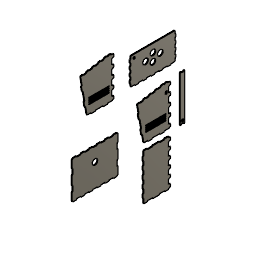
FINAL_CONSOLE (Autodesk Fusion 360 design; units mm, degrees)
part number: 2026-05-18-11-19-14-650
Autodesk Fusion 360 part; units mm, degrees
(part 1 of 2)
sketch "Sketch1" plane through (0, 0, 0) normal (1, 0, 0) x (0, 1, 0)
  line L0 (-1580.457, 35.3013) -> (-1610.457, 35.3013) construction
  line L1 (-1670.457, -232.1266) -> (-1670.457, -238.1266)
  line L2 (-1610.457, 43.2364) -> (-1580.457, 43.2364)
  line L3 (-1580.457, -232.1266) -> (-1574.457, -232.1266)
  line L4 (-1580.457, -22.7636) -> (-1574.457, -22.7636)
  line L5 (-1580.457, -232.1266) -> (-1580.457, 37.2364)
  line L6 (-1610.457, 37.2364) -> (-1610.457, 43.2364)
  line L7 (-1670.457, -238.1266) -> (-1640.457, -238.1266)
  line L8 (-1574.457, -232.1266) -> (-1574.457, -172.1266)
  line L9 (-1610.457, -232.1266) -> (-1610.457, -238.1266)
  line L10 (-1760.457, -232.1266) -> (-1760.457, -238.1266)
  line L11 (-1910.457, -232.1266) -> (-1580.457, -232.1266)
  line L12 (-1760.457, 43.2364) -> (-1790.457, 43.2364)
  line L13 (-1910.457, -232.1266) -> (-1580.457, -232.1266)
  line L14 (-1730.457, 37.2364) -> (-1730.457, 43.2364)
  line L15 (-1790.457, -238.1266) -> (-1760.457, -238.1266)
  line L16 (-1910.457, -232.1266) -> (-1580.457, -232.1266)
  line L17 (-1910.457, -232.1266) -> (-1580.457, -232.1266)
  circle A0 centre (-1745.457, -62.7636) radius 20
  line L18 (-1580.457, 37.2364) -> (-1910.457, 37.2364)
  line L19 (-1910.457, 37.2364) -> (-1910.457, -232.1266)
  line L20 (-1910.457, -172.1266) -> (-1916.457, -172.1266)
  line L21 (-1916.457, -22.7636) -> (-1916.457, 37.2364)
  line L22 (-1910.457, -22.7636) -> (-1916.457, -22.7636)
  line L23 (-1820.457, 37.2364) -> (-1820.457, 43.2364)
  line L24 (-1916.457, -132.1266) -> (-1916.457, -62.7636)
  line L25 (-1850.457, -232.1266) -> (-1850.457, -238.1266)
  line L26 (-1910.457, -238.1266) -> (-1880.457, -238.1266)
  line L27 (-1910.457, 37.2364) -> (-1910.457, 43.2364)
  line L28 (-1910.457, -62.7636) -> (-1916.457, -62.7636)
  line L29 (-1910.457, -232.1266) -> (-1910.457, -238.1266)
  line L30 (-1910.457, 43.2364) -> (-1880.457, 43.2364)
  line L31 (-1610.457, -238.1266) -> (-1580.457, -238.1266)
  line L32 (-1640.457, -232.1266) -> (-1640.457, -238.1266)
  line L33 (-1640.457, 43.2364) -> (-1670.457, 43.2364)
  line L34 (-1580.457, -232.1266) -> (-1580.457, -238.1266)
  line L35 (-1670.457, 37.2364) -> (-1670.457, 43.2364)
  line L36 (-1760.457, 37.2364) -> (-1760.457, 43.2364)
  line L37 (-1580.457, -172.1266) -> (-1574.457, -172.1266)
  line L38 (-1574.457, -132.1266) -> (-1574.457, -62.7636)
  line L39 (-1640.457, 37.2364) -> (-1640.457, 43.2364)
  line L40 (-1820.457, -232.1266) -> (-1820.457, -238.1266)
  line L41 (-1700.457, 43.2364) -> (-1730.457, 43.2364)
  line L42 (-1700.457, 37.2364) -> (-1700.457, 43.2364)
  line L43 (-1574.457, -22.7636) -> (-1574.457, 37.2364)
  line L44 (-1700.457, -232.1266) -> (-1700.457, -238.1266)
  line L45 (-1580.457, 37.2364) -> (-1574.457, 37.2364)
  line L46 (-1580.457, 37.2364) -> (-1580.457, 43.2364)
  line L47 (-1580.457, -132.1266) -> (-1574.457, -132.1266)
  line L48 (-1730.457, -232.1266) -> (-1730.457, -238.1266)
  line L49 (-1730.457, -238.1266) -> (-1700.457, -238.1266)
  line L50 (-1850.457, -238.1266) -> (-1820.457, -238.1266)
  line L51 (-1580.457, -62.7636) -> (-1574.457, -62.7636)
  line L52 (-1916.457, -232.1266) -> (-1916.457, -172.1266)
  line L53 (-1880.457, 43.2364) -> (-1880.457, 37.2364)
  line L54 (-1910.457, -232.1266) -> (-1916.457, -232.1266)
  line L55 (-1790.457, -232.1266) -> (-1790.457, -238.1266)
  line L56 (-1910.457, 37.2364) -> (-1916.457, 37.2364)
  line L57 (-1820.457, 43.2364) -> (-1850.457, 43.2364)
  line L58 (-1880.457, -232.1266) -> (-1880.457, -238.1266)
  line L59 (-1850.457, 37.2364) -> (-1850.457, 43.2364)
  line L60 (-1790.457, 37.2364) -> (-1790.457, 43.2364)
  line L61 (-1910.457, -132.1266) -> (-1916.457, -132.1266)
  line L62 (-1580.457, 35.3013) -> (-1610.457, 35.3013) construction
  line L63 (-1670.457, -232.1266) -> (-1670.457, -238.1266)
  line L64 (-1610.457, 43.2364) -> (-1580.457, 43.2364)
  line L65 (-1580.457, -232.1266) -> (-1574.457, -232.1266)
  line L66 (-1580.457, -22.7636) -> (-1574.457, -22.7636)
  line L67 (-1580.457, -232.1266) -> (-1580.457, 37.2364)
  line L68 (-1610.457, 37.2364) -> (-1610.457, 43.2364)
  line L69 (-1670.457, -238.1266) -> (-1640.457, -238.1266)
  line L70 (-1574.457, -232.1266) -> (-1574.457, -172.1266)
  line L71 (-1610.457, -232.1266) -> (-1610.457, -238.1266)
  line L72 (-1760.457, -232.1266) -> (-1760.457, -238.1266)
  line L73 (-1910.457, -232.1266) -> (-1580.457, -232.1266)
  line L74 (-1760.457, 43.2364) -> (-1790.457, 43.2364)
  line L75 (-1910.457, -232.1266) -> (-1580.457, -232.1266)
  line L76 (-1730.457, 37.2364) -> (-1730.457, 43.2364)
  line L77 (-1790.457, -238.1266) -> (-1760.457, -238.1266)
  line L78 (-1910.457, -232.1266) -> (-1580.457, -232.1266)
  line L79 (-1910.457, -232.1266) -> (-1580.457, -232.1266)
  circle A1 centre (-1745.457, -62.7636) radius 20
  line L80 (-1580.457, 37.2364) -> (-1910.457, 37.2364)
  line L81 (-1910.457, 37.2364) -> (-1910.457, -232.1266)
  line L82 (-1910.457, -172.1266) -> (-1916.457, -172.1266)
  line L83 (-1916.457, -22.7636) -> (-1916.457, 37.2364)
  line L84 (-1910.457, -22.7636) -> (-1916.457, -22.7636)
  line L85 (-1820.457, 37.2364) -> (-1820.457, 43.2364)
  line L86 (-1916.457, -132.1266) -> (-1916.457, -62.7636)
  line L87 (-1850.457, -232.1266) -> (-1850.457, -238.1266)
  line L88 (-1910.457, -238.1266) -> (-1880.457, -238.1266)
  line L89 (-1910.457, 37.2364) -> (-1910.457, 43.2364)
  line L90 (-1910.457, -62.7636) -> (-1916.457, -62.7636)
  line L91 (-1910.457, -232.1266) -> (-1910.457, -238.1266)
  line L92 (-1910.457, 43.2364) -> (-1880.457, 43.2364)
  line L93 (-1610.457, -238.1266) -> (-1580.457, -238.1266)
  line L94 (-1640.457, -232.1266) -> (-1640.457, -238.1266)
  line L95 (-1640.457, 43.2364) -> (-1670.457, 43.2364)
  line L96 (-1580.457, -232.1266) -> (-1580.457, -238.1266)
  line L97 (-1670.457, 37.2364) -> (-1670.457, 43.2364)
  line L98 (-1760.457, 37.2364) -> (-1760.457, 43.2364)
  line L99 (-1580.457, -172.1266) -> (-1574.457, -172.1266)
  line L100 (-1574.457, -132.1266) -> (-1574.457, -62.7636)
  line L101 (-1640.457, 37.2364) -> (-1640.457, 43.2364)
  line L102 (-1820.457, -232.1266) -> (-1820.457, -238.1266)
  line L103 (-1700.457, 43.2364) -> (-1730.457, 43.2364)
  line L104 (-1700.457, 37.2364) -> (-1700.457, 43.2364)
  line L105 (-1574.457, -22.7636) -> (-1574.457, 37.2364)
  line L106 (-1700.457, -232.1266) -> (-1700.457, -238.1266)
  line L107 (-1580.457, 37.2364) -> (-1574.457, 37.2364)
  line L108 (-1580.457, 37.2364) -> (-1580.457, 43.2364)
  line L109 (-1580.457, -132.1266) -> (-1574.457, -132.1266)
  line L110 (-1730.457, -232.1266) -> (-1730.457, -238.1266)
  line L111 (-1730.457, -238.1266) -> (-1700.457, -238.1266)
  line L112 (-1850.457, -238.1266) -> (-1820.457, -238.1266)
  line L113 (-1580.457, -62.7636) -> (-1574.457, -62.7636)
  line L114 (-1916.457, -232.1266) -> (-1916.457, -172.1266)
  line L115 (-1880.457, 43.2364) -> (-1880.457, 37.2364)
  line L116 (-1910.457, -232.1266) -> (-1916.457, -232.1266)
  line L117 (-1790.457, -232.1266) -> (-1790.457, -238.1266)
  line L118 (-1910.457, 37.2364) -> (-1916.457, 37.2364)
  line L119 (-1820.457, 43.2364) -> (-1850.457, 43.2364)
  line L120 (-1880.457, -232.1266) -> (-1880.457, -238.1266)
  line L121 (-1850.457, 37.2364) -> (-1850.457, 43.2364)
  line L122 (-1790.457, 37.2364) -> (-1790.457, 43.2364)
  line L123 (-1910.457, -132.1266) -> (-1916.457, -132.1266)
  line L124 (-1580.457, 35.3013) -> (-1610.457, 35.3013) construction
  line L125 (-1670.457, -232.1266) -> (-1670.457, -238.1266)
  line L126 (-1610.457, 43.2364) -> (-1580.457, 43.2364)
  line L127 (-1580.457, -232.1266) -> (-1574.457, -232.1266)
  line L128 (-1580.457, -22.7636) -> (-1574.457, -22.7636)
  line L129 (-1580.457, -232.1266) -> (-1580.457, 37.2364)
  line L130 (-1610.457, 37.2364) -> (-1610.457, 43.2364)
  line L131 (-1670.457, -238.1266) -> (-1640.457, -238.1266)
  line L132 (-1574.457, -232.1266) -> (-1574.457, -172.1266)
  line L133 (-1610.457, -232.1266) -> (-1610.457, -238.1266)
  line L134 (-1760.457, -232.1266) -> (-1760.457, -238.1266)
  line L135 (-1910.457, -232.1266) -> (-1580.457, -232.1266)
  line L136 (-1760.457, 43.2364) -> (-1790.457, 43.2364)
  line L137 (-1910.457, -232.1266) -> (-1580.457, -232.1266)
  line L138 (-1730.457, 37.2364) -> (-1730.457, 43.2364)
  line L139 (-1790.457, -238.1266) -> (-1760.457, -238.1266)
  line L140 (-1910.457, -232.1266) -> (-1580.457, -232.1266)
  line L141 (-1910.457, -232.1266) -> (-1580.457, -232.1266)
  circle A2 centre (-1745.457, -62.7636) radius 20
  line L142 (-1580.457, 37.2364) -> (-1910.457, 37.2364)
  line L143 (-1910.457, 37.2364) -> (-1910.457, -232.1266)
  line L144 (-1910.457, -172.1266) -> (-1916.457, -172.1266)
  line L145 (-1916.457, -22.7636) -> (-1916.457, 37.2364)
  line L146 (-1910.457, -22.7636) -> (-1916.457, -22.7636)
  line L147 (-1820.457, 37.2364) -> (-1820.457, 43.2364)
  line L148 (-1916.457, -132.1266) -> (-1916.457, -62.7636)
  line L149 (-1850.457, -232.1266) -> (-1850.457, -238.1266)
  line L150 (-1910.457, -238.1266) -> (-1880.457, -238.1266)
  line L151 (-1910.457, 37.2364) -> (-1910.457, 43.2364)
  line L152 (-1910.457, -62.7636) -> (-1916.457, -62.7636)
  line L153 (-1910.457, -232.1266) -> (-1910.457, -238.1266)
  line L154 (-1910.457, 43.2364) -> (-1880.457, 43.2364)
  line L155 (-1610.457, -238.1266) -> (-1580.457, -238.1266)
  line L156 (-1640.457, -232.1266) -> (-1640.457, -238.1266)
  line L157 (-1640.457, 43.2364) -> (-1670.457, 43.2364)
  line L158 (-1580.457, -232.1266) -> (-1580.457, -238.1266)
  line L159 (-1670.457, 37.2364) -> (-1670.457, 43.2364)
  line L160 (-1760.457, 37.2364) -> (-1760.457, 43.2364)
  line L161 (-1580.457, -172.1266) -> (-1574.457, -172.1266)
  line L162 (-1574.457, -132.1266) -> (-1574.457, -62.7636)
  line L163 (-1640.457, 37.2364) -> (-1640.457, 43.2364)
  line L164 (-1820.457, -232.1266) -> (-1820.457, -238.1266)
  line L165 (-1700.457, 43.2364) -> (-1730.457, 43.2364)
  line L166 (-1700.457, 37.2364) -> (-1700.457, 43.2364)
  line L167 (-1574.457, -22.7636) -> (-1574.457, 37.2364)
  line L168 (-1700.457, -232.1266) -> (-1700.457, -238.1266)
  line L169 (-1580.457, 37.2364) -> (-1574.457, 37.2364)
  line L170 (-1580.457, 37.2364) -> (-1580.457, 43.2364)
  line L171 (-1580.457, -132.1266) -> (-1574.457, -132.1266)
  line L172 (-1730.457, -232.1266) -> (-1730.457, -238.1266)
  line L173 (-1730.457, -238.1266) -> (-1700.457, -238.1266)
  line L174 (-1850.457, -238.1266) -> (-1820.457, -238.1266)
  line L175 (-1580.457, -62.7636) -> (-1574.457, -62.7636)
  line L176 (-1916.457, -232.1266) -> (-1916.457, -172.1266)
  line L177 (-1880.457, 43.2364) -> (-1880.457, 37.2364)
  line L178 (-1910.457, -232.1266) -> (-1916.457, -232.1266)
  line L179 (-1790.457, -232.1266) -> (-1790.457, -238.1266)
  line L180 (-1910.457, 37.2364) -> (-1916.457, 37.2364)
  line L181 (-1820.457, 43.2364) -> (-1850.457, 43.2364)
  line L182 (-1880.457, -232.1266) -> (-1880.457, -238.1266)
  line L183 (-1850.457, 37.2364) -> (-1850.457, 43.2364)
  line L184 (-1790.457, 37.2364) -> (-1790.457, 43.2364)
  line L185 (-1910.457, -132.1266) -> (-1916.457, -132.1266)
  line L186 (-1103.0897, 195.8237) -> (-1113.0897, 195.8237)
  line L187 (-1390.0582, 280.2873) -> (-1360.0582, 280.2873)
  line L188 (-1360.0582, 280.2873) -> (-1360.0582, 286.2873)
  line L189 (-1847.5452, 473.2585) -> (-1840.5992, 433.8662)
  line L190 (-1233.3072, 178.4245) -> (-1198.3072, 178.4245)
  line L191 (-1192.3072, 178.4245) -> (-1192.3072, 173.4245)
  line L192 (-1192.3306, 85.9666) -> (-1183.3306, 85.9666)
  line L193 (-1809.2732, 547.0251) -> (-1787.6074, 550.8453)
  line L194 (-1360.0582, 280.2873) -> (-1360.0582, 286.2873)
  line L195 (-1192.3306, 110.9666) -> (-1198.3306, 110.9666)
  line L196 (-1198.3072, 80.9667) -> (-1192.3072, 80.9667)
  line L197 (-1209.8072, 109.4245) -> (-1221.8072, 109.4245)
  line L198 (-1183.3306, 105.9666) -> (-1192.3306, 105.9666)
  line L199 (-1210.0582, 286.2873) -> (-1210.0582, 280.2873)
  line L200 (-1210.0582, 286.2873) -> (-1210.0582, 280.2873)
  line L201 (-1330.0582, 286.2873) -> (-1330.0582, 280.2873)
  line L202 (-1192.9109, -362.5837) -> (-1192.8771, -357.8609)
  line L203 (-1144.0942, 331.3501) -> (-1144.086, 308.8501)
  line L204 (-1480.0582, 464.2873) -> (-1486.0582, 464.2873)
  line L205 (-1486.0582, 441.7873) -> (-1480.0582, 441.7873)
  circle A3 centre (-1315.0582, 426.2873) radius 20
  line L206 (-1189.9109, -502.5837) -> (-1183.9109, -502.5837)
  line L207 (-1210.0582, 280.2873) -> (-1180.0582, 280.2873)
  line L208 (-1150.1023, 486.3479) -> (-1150.0892, 450.6275)
  line L209 (-1150.0942, 420.0146) -> (-1144.0942, 420.0168)
  line L210 (-1390.0582, 280.2873) -> (-1360.0582, 280.2873)
  line L211 (-1330.0582, 286.2873) -> (-1330.0582, 280.2873)
  line L212 (-1721.6253, 562.4798) -> (-1699.9595, 566.3)
  line L213 (-1486.0582, 308.2873) -> (-1480.0582, 308.2873)
  line L214 (-1150.0942, 464.3479) -> (-1144.0942, 464.3501)
  line L215 (-1192.3072, 148.4245) -> (-1198.3072, 148.4245)
  line L216 (-1330.0582, 280.2873) -> (-1300.0582, 280.2873)
  line L217 (-1180.0582, 280.2873) -> (-1180.0582, 286.2873)
  line L218 (-1210.0582, 286.2873) -> (-1210.0582, 280.2873)
  line L219 (-1300.0582, 280.2873) -> (-1300.0582, 286.2873)
  line L220 (-1150.1023, 353.3479) -> (-1150.0892, 317.6275)
  line L221 (-1330.0582, 280.2873) -> (-1300.0582, 280.2873)
  line L222 (-1480.0582, 375.2873) -> (-1486.0582, 375.2873)
  line L223 (-1486.0582, 397.2873) -> (-1480.0582, 397.2873)
  line L224 (-1183.3072, 173.4245) -> (-1183.3072, 153.4245)
  line L225 (-1180.0582, 280.2873) -> (-1180.0582, 286.2873)
  line L226 (-1210.0582, 280.2873) -> (-1180.0582, 280.2873)
  line L227 (-1103.0897, 189.8237) -> (-1103.0897, 195.8237)
  line L228 (-1300.0582, 280.2873) -> (-1300.0582, 286.2873)
  circle A4 centre (-1455.0582, 461.2873) radius 8
  line L229 (-1742.7416, 552.6638) -> (-1743.7834, 558.5727)
  line L230 (-1330.0582, 280.2873) -> (-1300.0582, 280.2873)
  line L231 (-1221.8072, 128.4245) -> (-1209.8072, 128.4245)
  line L232 (-1330.0582, 280.2873) -> (-1300.0582, 280.2873)
  line L233 (-1486.0582, 419.7873) -> (-1486.0582, 397.2873)
  line L234 (-1330.0582, 286.2873) -> (-1330.0582, 280.2873)
  line L235 (-1486.0582, 352.7873) -> (-1480.0582, 352.7873)
  line L236 (-1144.0942, 464.3501) -> (-1144.086, 441.8501)
  line L237 (-1144.0942, 420.0168) -> (-1144.086, 397.5168)
  line L238 (-1192.9109, -482.5837) -> (-1192.9109, -477.5837)
  line L239 (-1210.0582, 286.2873) -> (-1210.0582, 280.2873)
  line L240 (-1480.0582, 486.2873) -> (-1480.0582, 450.5669)
  line L241 (-1330.0582, 286.2873) -> (-1330.0582, 280.2873)
  line L242 (-1198.9416, -447.7821) -> (-1192.9417, -447.8176)
  line L243 (-1210.0582, 280.2873) -> (-1180.0582, 280.2873)
  line L244 (-1192.3072, 80.9667) -> (-1192.3306, 85.9666)
  line L245 (-1840.5992, 433.8662) -> (-1834.6904, 434.9081)
  circle A5 centre (-1315.0582, 366.2873) radius 20
  line L246 (-1223.3072, 184.4245) -> (-1208.3072, 184.4245)
  line L247 (-1180.0582, 280.2873) -> (-1180.0582, 286.2873)
  line L248 (-1180.0582, 280.2873) -> (-1180.0582, 286.2873)
  line L249 (-1330.0582, 280.2873) -> (-1300.0582, 280.2873)
  line L250 (-1113.0897, 189.8237) -> (-1078.0897, 189.8237)
  line L251 (-1103.0897, -140.1763) -> (-1103.0897, -146.1763)
  line L252 (-1808.2313, 541.1162) -> (-1809.2732, 547.0251)
  line L253 (-1144.0942, 375.6834) -> (-1144.086, 353.1834)
  line L254 (-1218.3072, -55.6009) -> (-1218.3072, -60.6009)
  line L255 (-1150.1023, 442.0146) -> (-1150.0892, 406.2941)
  line L256 (-1210.0582, 280.2873) -> (-1180.0582, 280.2873)
  line L257 (-1192.9461, -387.8486) -> (-1192.9109, -382.5837)
  line L258 (-1210.0582, 286.2873) -> (-1210.0582, 280.2873)
  line L259 (-1183.3306, -28.9524) -> (-1192.3306, -28.9524)
  line L260 (-1144.086, 353.1834) -> (-1150.086, 353.1812)
  line L261 (-1210.0582, 280.2873) -> (-1180.0582, 280.2873)
  line L262 (-1150.0942, 375.6812) -> (-1144.0942, 375.6834)
  line L263 (-1480.0582, 419.7873) -> (-1486.0582, 419.7873)
  line L264 (-1144.086, 308.8501) -> (-1150.086, 308.8479)
  line L265 (-1480.0582, 330.7873) -> (-1486.0582, 330.7873)
  line L266 (-1078.0897, -140.1763) -> (-1078.0897, -146.1763)
  line L267 (-1192.3306, -28.9524) -> (-1192.3306, -23.9524)
  line L268 (-1830.3894, 537.2091) -> (-1831.4313, 543.118)
  line L269 (-1210.0582, 286.2873) -> (-1210.0582, 280.2873)
  line L270 (-1183.9109, -362.5837) -> (-1192.9109, -362.5837)
  line L271 (-1180.0582, 280.2873) -> (-1180.0582, 286.2873)
  line L272 (-1210.0582, 280.2873) -> (-1180.0582, 280.2873)
  line L273 (-1144.086, 397.5168) -> (-1150.086, 397.5146)
  circle A6 centre (-1370.0582, 396.2873) radius 20
  line L274 (-1144.086, 441.8501) -> (-1150.086, 441.8479)
  circle A7 centre (-1260.0582, 396.2873) radius 20
  line L275 (-1486.0582, 330.7873) -> (-1486.0582, 308.2873)
  line L276 (-1180.0582, 280.2873) -> (-1180.0582, 286.2873)
  line L277 (-1150.1023, 397.6812) -> (-1150.0892, 361.9608)
  line L278 (-1486.0582, 375.2873) -> (-1486.0582, 352.7873)
  line L279 (-1330.0582, 280.2873) -> (-1300.0582, 280.2873)
  line L280 (-1330.0582, 286.2873) -> (-1330.0582, 280.2873)
  line L281 (-1486.0582, 464.2873) -> (-1486.0582, 441.7873)
  line L282 (-1853.0971, 539.2977) -> (-1831.4313, 543.118)
  line L283 (-1198.9459, -387.8085) -> (-1192.9461, -387.8486)
  line L284 (-1330.0582, 280.2873) -> (-1300.0582, 280.2873)
  line L285 (-1180.0582, 280.2873) -> (-1180.0582, 286.2873)
  line L286 (-1150.0942, 331.3479) -> (-1144.0942, 331.3501)
  line L287 (-1210.0582, 280.2873) -> (-1180.0582, 280.2873)
  line L288 (-1852.0552, 533.3889) -> (-1853.0971, 539.2977)
  line L289 (-1384.0979, -177.5837) -> (-1384.0979, -171.5837)
  line L290 (-1318.4944, -127.5755) -> (-1318.4944, -121.5755)
  line L291 (-1354.0979, -177.5837) -> (-1354.0979, -171.5837)
  line L292 (-1218.3072, -15.6009) -> (-1218.3072, -20.6009)
  line L293 (-1419.8499, 84.6064) -> (-1425.7587, 83.5645)
  line L294 (-1218.3072, -47.2676) -> (-1368.3072, -47.2676)
  line L295 (-1390.0979, -267.5837) -> (-1390.0979, -297.5837)
  line L296 (-1450.0582, 280.2873) -> (-1420.0582, 280.2873)
  line L297 (-1390.0979, -327.5837) -> (-1390.0979, -357.5837)
  line L298 (-1384.0979, -507.5837) -> (-1384.0979, -177.5837)
  line L299 (-1368.3072, -20.6009) -> (-1368.3072, -15.6009)
  line L300 (-1319.0979, -177.5837) -> (-1319.0979, -171.5837)
  line L301 (-1263.9109, -171.5837) -> (-1319.0979, -171.5837)
  line L302 (-1390.0979, -297.5837) -> (-1384.0979, -297.5837)
  line L303 (-1420.0582, 280.2873) -> (-1420.0582, 286.2873)
  line L304 (-1450.0582, 280.2873) -> (-1420.0582, 280.2873)
  line L305 (-1450.0582, 286.2873) -> (-1450.0582, 280.2873)
  line L306 (-1218.3072, -20.6009) -> (-1368.3072, -20.6009)
  line L307 (-1256.0149, 180.5131) -> (-1234.3491, 184.3333)
  line L308 (-1390.0979, -207.5837) -> (-1390.0979, -237.5837)
  line L309 (-1384.0979, -327.5837) -> (-1390.0979, -327.5837)
  line L310 (-1384.0979, -267.5837) -> (-1390.0979, -267.5837)
  line L311 (-1420.0582, 280.2873) -> (-1420.0582, 286.2873)
  line L312 (-1198.9109, -177.5837) -> (-1198.9109, -507.5837)
  line L313 (-1620.0937, 568.1185) -> (-1620.0937, 268.2822)
  line L314 (-1228.3072, -121.5521) -> (-1228.3072, -127.5755)
  line L315 (-1430.2687, 143.6949) -> (-1383.4944, -121.5755)
  line L316 (-1852.0552, 533.3889) -> (-1805.2809, 268.1185)
  line L317 (-1384.0979, -507.5837) -> (-1195.9109, -507.5837)
  line L318 (-1233.3072, 178.4245) -> (-1234.3491, 184.3333)
  line L319 (-1384.0979, -207.5837) -> (-1390.0979, -207.5837)
  line L320 (-1384.0979, -507.5837) -> (-1198.9109, -507.5837)
  line L321 (-1390.0582, 286.2873) -> (-1390.0582, 280.2873)
  line L322 (-1263.9109, -177.5837) -> (-1263.9109, -171.5837)
  line L323 (-1431.3106, 149.6037) -> (-1409.6449, 153.424)
  line L324 (-1390.0582, 286.2873) -> (-1390.0582, 280.2873)
  line L325 (-1277.1311, 170.6971) -> (-1278.173, 176.606)
  line L326 (-1354.0979, -171.5837) -> (-1384.0979, -171.5837)
  line L327 (-1390.0582, 286.2873) -> (-1390.0582, 280.2873)
  line L328 (-1368.3072, -47.2676) -> (-1368.3072, -42.2676)
  line L329 (-1425.7587, 83.5645) -> (-1418.8128, 44.1722)
  line L330 (-1198.9109, -507.5837) -> (-1384.0979, -507.5837)
  line L331 (-1368.3072, -28.9343) -> (-1218.3072, -28.9343)
  line L332 (-1390.0979, -237.5837) -> (-1384.0979, -237.5837)
  line L333 (-1450.0582, 286.2873) -> (-1450.0582, 280.2873)
  line L334 (-1387.4867, 157.331) -> (-1365.8209, 161.1513)
  line L335 (-1450.0582, 280.2873) -> (-1420.0582, 280.2873)
  line L336 (-1218.3072, -33.9343) -> (-1368.3072, -33.9343)
  line L337 (-1368.3072, -55.6009) -> (-1218.3072, -55.6009)
  line L338 (-1614.0937, 365.74) -> (-1614.0937, 360.74)
  line L339 (-1320.9551, 162.9698) -> (-1321.997, 168.8786)
  line L340 (-1368.3072, -15.6009) -> (-1218.3072, -15.6009)
  line L341 (-1450.0582, 286.2873) -> (-1450.0582, 280.2873)
  line L342 (-1450.0582, 280.2873) -> (-1420.0582, 280.2873)
  line L343 (-1342.6209, 159.1495) -> (-1343.6627, 165.0584)
  line L344 (-1150.0582, 486.2873) -> (-1480.0582, 486.2873)
  line L345 (-1685.0937, 262.1185) -> (-1685.0937, 268.1185)
  line L346 (-1263.9109, -513.5837) -> (-1319.0979, -513.5837)
  line L347 (-1450.0582, 286.2873) -> (-1450.0582, 280.2873)
  line L348 (-1480.0582, 486.2873) -> (-1150.0582, 486.2873)
  line L349 (-1640.0937, 347.4264) -> (-1640.0937, 342.4264)
  line L350 (-1406.7681, -24.1366) -> (-1400.8592, -23.0947)
  line L351 (-1450.0582, 280.2873) -> (-1420.0582, 280.2873)
  line L352 (-1384.0979, -507.5837) -> (-1384.0979, -513.5837)
  line L353 (-1218.3072, -28.9343) -> (-1218.3072, -33.9343)
  line L354 (-1384.0979, -447.5837) -> (-1390.0979, -447.5837)
  line L355 (-1354.0979, -507.5837) -> (-1354.0979, -513.5837)
  line L356 (-1420.0582, 280.2873) -> (-1420.0582, 286.2873)
  line L357 (-1418.8128, 44.1722) -> (-1412.9039, 45.2141)
  line L358 (-1420.0582, 280.2873) -> (-1420.0582, 286.2873)
  line L359 (-1605.0937, 293.2805) -> (-1605.0937, 273.2805)
  line L360 (-1150.0582, 286.2873) -> (-1480.0582, 286.2873)
  line L361 (-1354.0979, -513.5837) -> (-1384.0979, -513.5837)
  line L362 (-1420.0582, 280.2873) -> (-1420.0582, 286.2873)
  line L363 (-1614.0937, 293.2805) -> (-1605.0937, 293.2805)
  line L364 (-1353.4944, -127.5755) -> (-1318.4944, -127.5755)
  line L365 (-1614.0937, 268.2805) -> (-1620.0937, 268.2822)
  line L366 (-1218.3072, -60.6009) -> (-1368.3072, -60.6009)
  line L367 (-1390.0582, 286.2873) -> (-1390.0582, 280.2873)
  line L368 (-1605.0937, 340.74) -> (-1614.0937, 340.74)
  line L369 (-1430.2687, 143.6949) -> (-1431.3106, 149.6037)
  line L370 (-1195.9109, -507.5837) -> (-1189.9109, -507.5837)
  line L371 (-1192.9109, -422.5837) -> (-1192.8811, -417.8271)
  line L372 (-1298.7969, 166.8769) -> (-1299.8388, 172.7857)
  line L373 (-1198.9109, -513.5837) -> (-1228.9109, -513.5837)
  line L374 (-1183.9109, -242.5837) -> (-1192.9109, -242.5837)
  line L375 (-1263.3072, -127.5755) -> (-1263.3072, -121.5755)
  line L376 (-1450.0582, 280.2873) -> (-1420.0582, 280.2873)
  line L377 (-1368.3072, -42.2676) -> (-1218.3072, -42.2676)
  line L378 (-1192.9109, -182.5837) -> (-1192.8541, -178.0547)
  line L379 (-1390.0979, -417.5837) -> (-1384.0979, -417.5837)
  line L380 (-1650.0937, 268.1419) -> (-1650.0937, 262.1185)
  line L381 (-1384.0979, -387.5837) -> (-1390.0979, -387.5837)
  line L382 (-1614.0937, 298.2805) -> (-1620.0937, 298.2805)
  line L383 (-1300.0582, 280.2873) -> (-1300.0582, 286.2873)
  line L384 (-1088.0897, 189.8237) -> (-1088.0897, 195.8237)
  line L385 (-1390.0582, 280.2873) -> (-1360.0582, 280.2873)
  line L386 (-1209.8072, 128.4245) -> (-1209.8072, 109.4245)
  line L387 (-1841.6363, 474.3004) -> (-1847.5452, 473.2585)
  line L388 (-1300.0582, 280.2873) -> (-1300.0582, 286.2873)
  line L389 (-1390.0582, 280.2873) -> (-1360.0582, 280.2873)
  line L390 (-1330.0582, 280.2873) -> (-1300.0582, 280.2873)
  line L391 (-1330.0582, 286.2873) -> (-1330.0582, 280.2873)
  line L392 (-1183.3306, 85.9666) -> (-1183.3306, 105.9666)
  line L393 (-1360.0582, 280.2873) -> (-1360.0582, 286.2873)
  line L394 (-1720.5834, 556.5709) -> (-1721.6253, 562.4798)
  line L395 (-1192.3306, 105.9666) -> (-1192.3306, 110.9666)
  line L396 (-1390.0582, 280.2873) -> (-1360.0582, 280.2873)
  line L397 (-1192.9109, -442.5837) -> (-1183.9109, -442.5837)
  line L398 (-1300.0582, 280.2873) -> (-1300.0582, 286.2873)
  line L399 (-1198.3072, 178.4245) -> (-1192.3072, 178.4245)
  line L400 (-1210.0582, 286.2873) -> (-1210.0582, 280.2873)
  line L401 (-1078.0897, 189.8237) -> (-1078.0897, 195.8237)
  line L402 (-1764.4073, 548.8436) -> (-1765.4492, 554.7524)
  line L403 (-1180.0582, 280.2873) -> (-1180.0582, 286.2873)
  line L404 (-1300.0582, 280.2873) -> (-1300.0582, 286.2873)
  line L405 (-1300.0582, 280.2873) -> (-1300.0582, 286.2873)
  line L406 (-1210.0582, 280.2873) -> (-1180.0582, 280.2873)
  line L407 (-1786.5655, 544.9365) -> (-1787.6074, 550.8453)
  line L408 (-1192.8811, -417.8271) -> (-1198.9109, -417.8271)
  line L409 (-1208.3072, 184.4245) -> (-1208.3072, 178.4245)
  line L410 (-1330.0582, 286.2873) -> (-1330.0582, 280.2873)
  line L411 (-1390.0582, 280.2873) -> (-1360.0582, 280.2873)
  line L412 (-1113.0897, 189.8237) -> (-1113.0897, 195.8237)
  line L413 (-1300.0582, 280.2873) -> (-1300.0582, 286.2873)
  line L414 (-1360.0582, 280.2873) -> (-1360.0582, 286.2873)
  line L415 (-1765.4492, 554.7524) -> (-1743.7834, 558.5727)
  line L416 (-1183.3072, 153.4245) -> (-1192.3072, 153.4245)
  line L417 (-1192.3072, 173.4245) -> (-1183.3072, 173.4245)
  line L418 (-1183.9109, -422.5837) -> (-1192.9109, -422.5837)
  line L419 (-1078.0897, 195.8237) -> (-1088.0897, 195.8237)
  line L420 (-1360.0582, 280.2873) -> (-1360.0582, 286.2873)
  line L421 (-1698.9176, 560.3912) -> (-1699.9595, 566.3)
  line L422 (-1183.9109, -482.5837) -> (-1183.9109, -502.5837)
  line L423 (-1192.3072, 153.4245) -> (-1192.3072, 148.4245)
  line L424 (-1330.0582, 286.2873) -> (-1330.0582, 280.2873)
  line L425 (-1614.0937, 563.1185) -> (-1605.0937, 563.1185)
  line L426 (-1360.0582, 280.2873) -> (-1360.0582, 286.2873)
  line L427 (-1360.0582, 280.2873) -> (-1360.0582, 286.2873)
  line L428 (-1828.5546, 365.5574) -> (-1822.6457, 366.5993)
  line L429 (-1088.0897, -140.1763) -> (-1088.0897, -146.1763)
  line L430 (-1790.0937, 342.4264) -> (-1790.0937, 347.4264)
  line L431 (-1270.0582, 280.2873) -> (-1240.0582, 280.2873)
  line L432 (-1198.9711, -207.9552) -> (-1192.9714, -208.0216)
  line L433 (-1390.0582, 280.2873) -> (-1360.0582, 280.2873)
  line L434 (-1790.0937, 355.7597) -> (-1790.0937, 360.7597)
  line L435 (-1192.9109, -382.5837) -> (-1183.9109, -382.5837)
  line L436 (-1270.0582, 286.2873) -> (-1270.0582, 280.2873)
  line L437 (-1655.0937, 568.1185) -> (-1674.2514, 564.7405) construction
  line L438 (-1192.9109, -262.5837) -> (-1183.9109, -262.5837)
  line L439 (-1270.0582, 280.2873) -> (-1240.0582, 280.2873)
  line L440 (-1815.6998, 327.207) -> (-1821.6086, 326.1651)
  line L441 (-1183.9109, -302.5837) -> (-1192.9109, -302.5837)
  line L442 (-1198.3072, -53.9523) -> (-1192.3072, -53.9523)
  line L443 (-1192.3306, 18.5071) -> (-1183.3306, 18.5071)
  line L444 (-1198.3072, -121.4118) -> (-1192.3072, -121.4118)
  line L445 (-1790.0937, 369.0931) -> (-1790.0937, 374.0931)
  line L446 (-1645.0937, 568.1185) -> (-1645.0937, 574.1185)
  line L447 (-1384.0979, -177.5837) -> (-1198.9109, -177.5837)
  line L448 (-1390.0582, 280.2873) -> (-1360.0582, 280.2873)
  line L449 (-1192.3306, 43.5071) -> (-1198.3306, 43.5071)
  line L450 (-1192.3072, 13.5072) -> (-1192.3306, 18.5071)
  line L451 (-1614.0937, 408.1995) -> (-1614.0937, 403.1995)
  line L452 (-1790.0937, 329.0931) -> (-1790.0937, 334.0931)
  line L453 (-1740.2809, 262.1185) -> (-1740.2809, 268.1185)
  line L454 (-1605.0937, 543.1185) -> (-1614.0937, 543.1185)
  line L455 (-1228.9109, -507.5837) -> (-1228.9109, -513.5837)
  line L456 (-1614.0937, 470.659) -> (-1620.0937, 470.659)
  line L457 (-1775.2809, 268.1185) -> (-1775.2809, 262.1185)
  line L458 (-1270.0582, 286.2873) -> (-1270.0582, 280.2873)
  line L459 (-1384.0979, -177.5837) -> (-1198.9109, -177.5837)
  line L460 (-1192.3072, -121.4118) -> (-1192.3306, -116.4119)
  line L461 (-1240.0582, 280.2873) -> (-1240.0582, 286.2873)
  line L462 (-1605.0937, 428.1995) -> (-1605.0937, 408.1995)
  line L463 (-1270.0582, 286.2873) -> (-1270.0582, 280.2873)
  line L464 (-1270.0582, 286.2873) -> (-1270.0582, 280.2873)
  line L465 (-1192.9109, -477.5837) -> (-1198.9109, -477.5837)
  line L466 (-1150.0582, 486.2873) -> (-1150.0582, 286.2873)
  line L467 (-1614.0937, 495.659) -> (-1605.0937, 495.659)
  line L468 (-1790.0937, 374.0931) -> (-1640.0937, 374.0931)
  line L469 (-1240.0582, 280.2873) -> (-1240.0582, 286.2873)
  line L470 (-1192.3306, -116.4119) -> (-1183.3306, -116.4119)
  line L471 (-1192.3306, -48.9524) -> (-1183.3306, -48.9524)
  line L472 (-1640.0937, 355.7597) -> (-1790.0937, 355.7597)
  line L473 (-1640.0937, 342.4264) -> (-1790.0937, 342.4264)
  line L474 (-1103.0897, -146.1763) -> (-1113.0897, -146.1763)
  line L475 (-1078.0897, 189.8237) -> (-1078.0897, -140.1763)
  line L476 (-1192.3306, 38.5071) -> (-1192.3306, 43.5071)
  line L477 (-1620.0937, 568.1185) -> (-1614.0937, 568.1185)
  line L478 (-1270.0582, 280.2873) -> (-1240.0582, 280.2873)
  line L479 (-1614.0937, 428.1995) -> (-1605.0937, 428.1995)
  line L480 (-1790.0937, 360.7597) -> (-1640.0937, 360.7597)
  line L481 (-1614.0937, 538.1185) -> (-1620.0937, 538.1185)
  line L482 (-1270.0582, 280.2873) -> (-1240.0582, 280.2873)
  line L483 (-1640.0937, 329.0931) -> (-1790.0937, 329.0931)
  line L484 (-1183.9109, -362.5837) -> (-1183.9109, -382.5837)
  line L485 (-1240.0582, 280.2873) -> (-1240.0582, 286.2873)
  line L486 (-1078.0897, -140.1763) -> (-1113.0897, -140.1763)
  line L487 (-1270.0582, 286.2873) -> (-1270.0582, 280.2873)
  line L488 (-1614.0937, 543.1185) -> (-1614.0937, 538.1185)
  line L489 (-1655.0937, 568.1185) -> (-1656.1356, 574.0274)
  line L490 (-1640.0937, 369.0931) -> (-1790.0937, 369.0931)
  line L491 (-1270.0582, 286.2873) -> (-1270.0582, 280.2873)
  line L492 (-1240.0582, 280.2873) -> (-1240.0582, 286.2873)
  line L493 (-1605.0937, 408.1995) -> (-1614.0937, 408.1995)
  line L494 (-1270.0582, 280.2873) -> (-1240.0582, 280.2873)
  line L495 (-1677.8013, 570.2071) -> (-1656.1356, 574.0274)
  line L496 (-1198.3072, 13.5072) -> (-1192.3072, 13.5072)
  line L497 (-1192.3306, -23.9524) -> (-1198.3306, -23.9524)
  line L498 (-1198.3072, -121.4118) -> (-1233.3072, -121.5755)
  line L499 (-1198.3072, 178.4245) -> (-1198.3072, -121.4118)
  line L500 (-1189.9109, -507.5837) -> (-1189.9109, -502.5837)
  line L501 (-1113.0897, -140.1763) -> (-1113.0897, -146.1763)
  line L502 (-1614.0937, 433.1995) -> (-1614.0937, 428.1995)
  line L503 (-1240.0582, 280.2873) -> (-1240.0582, 286.2873)
  line L504 (-1614.0937, 403.1995) -> (-1620.0937, 403.1995)
  line L505 (-1240.0582, 280.2873) -> (-1240.0582, 286.2873)
  line L506 (-1614.0937, 475.659) -> (-1614.0937, 470.659)
  line L507 (-1183.3306, -96.4119) -> (-1192.3306, -96.4119)
  line L508 (-1240.0582, 280.2873) -> (-1240.0582, 286.2873)
  line L509 (-1113.0897, -140.1763) -> (-1113.0897, 189.8237)
  line L510 (-1183.9109, -482.5837) -> (-1192.9109, -482.5837)
  line L511 (-1183.3306, -48.9524) -> (-1183.3306, -28.9524)
  line L512 (-1218.3072, -42.2676) -> (-1218.3072, -47.2676)
  line L513 (-1183.3306, 38.5071) -> (-1192.3306, 38.5071)
  line L514 (-1183.3306, 18.5071) -> (-1183.3306, 38.5071)
  line L515 (-1183.9109, -422.5837) -> (-1183.9109, -442.5837)
  line L516 (-1078.0897, -146.1763) -> (-1088.0897, -146.1763)
  line L517 (-1183.3306, -116.4119) -> (-1183.3306, -96.4119)
  line L518 (-1210.0582, 286.2873) -> (-1210.0582, 280.2873)
  line L519 (-1192.8771, -357.8609) -> (-1198.9109, -357.8609)
  line L520 (-1192.3306, -91.4119) -> (-1198.3306, -91.4119)
  line L521 (-1192.9109, -202.5837) -> (-1183.9109, -202.5837)
  line L522 (-1263.9109, -507.5837) -> (-1263.9109, -513.5837)
  line L523 (-1150.0582, 286.2873) -> (-1480.0582, 286.2873)
  line L524 (-1790.0937, 347.4264) -> (-1640.0937, 347.4264)
  line L525 (-1399.8222, -63.5289) -> (-1406.7681, -24.1366)
  line L526 (-1192.9417, -447.8176) -> (-1192.9109, -442.5837)
  line L527 (-1390.0582, 286.2873) -> (-1390.0582, 280.2873)
  line L528 (-1408.603, 147.5151) -> (-1409.6449, 153.424)
  line L529 (-1183.9109, -182.5837) -> (-1192.9109, -182.5837)
  line L530 (-1420.0582, 280.2873) -> (-1420.0582, 286.2873)
  line L531 (-1650.0937, 262.1185) -> (-1685.0937, 262.1185)
  line L532 (-1198.9516, -327.8427) -> (-1192.9518, -327.889)
  line L533 (-1353.4944, -121.5755) -> (-1353.4944, -127.5755)
  line L534 (-1390.0979, -357.5837) -> (-1384.0979, -357.5837)
  line L535 (-1390.0979, -447.5837) -> (-1390.0979, -477.5837)
  line L536 (-1390.0979, -387.5837) -> (-1390.0979, -417.5837)
  line L537 (-1620.0937, 268.2822) -> (-1655.0937, 268.1185)
  line L538 (-1420.0582, 280.2873) -> (-1420.0582, 286.2873)
  line L539 (-1614.0937, 335.74) -> (-1620.0937, 335.74)
  line L540 (-1383.4944, -121.5755) -> (-1233.3072, -121.5755)
  line L541 (-1450.0582, 286.2873) -> (-1450.0582, 280.2873)
  line L542 (-1198.9109, -171.5837) -> (-1228.9109, -171.5837)
  line L543 (-1640.0937, 360.7597) -> (-1640.0937, 355.7597)
  line L544 (-1614.0937, 340.74) -> (-1614.0937, 335.74)
  line L545 (-1192.9109, -322.5837) -> (-1183.9109, -322.5837)
  line L546 (-1192.8646, -237.9663) -> (-1198.9109, -237.9663)
  line L547 (-1605.0937, 360.74) -> (-1605.0937, 340.74)
  line L548 (-1364.779, 155.2425) -> (-1365.8209, 161.1513)
  line L549 (-1319.0979, -507.5837) -> (-1319.0979, -513.5837)
  line L550 (-1390.0979, -477.5837) -> (-1384.0979, -477.5837)
  line L551 (-1221.8072, 109.4245) -> (-1221.8072, 128.4245)
  line L552 (-1390.0582, 286.2873) -> (-1390.0582, 280.2873)
  line L553 (-1450.0582, 286.2873) -> (-1450.0582, 280.2873)
  line L554 (-1192.9518, -327.889) -> (-1192.9109, -322.5837)
  line L555 (-1655.0937, 568.1185) -> (-1852.0552, 533.3889)
  line L556 (-1223.3072, 178.4245) -> (-1223.3072, 184.4245)
  line L557 (-1390.0582, 286.2873) -> (-1390.0582, 280.2873)
  line L558 (-1254.973, 174.6042) -> (-1256.0149, 180.5131)
  line L559 (-1640.0937, 334.0931) -> (-1640.0937, 329.0931)
  line L560 (-1805.2809, 268.1185) -> (-1655.0937, 268.1185)
  line L561 (-1420.0582, 280.2873) -> (-1420.0582, 286.2873)
  line L562 (-1614.0937, 298.2805) -> (-1614.0937, 293.2805)
  line L563 (-1192.9109, -302.5837) -> (-1192.8718, -297.9053)
  line L564 (-1480.0582, 286.2873) -> (-1480.0582, 486.2873)
  line L565 (-1390.0582, 286.2873) -> (-1390.0582, 280.2873)
  line L566 (-1790.0937, 334.0931) -> (-1640.0937, 334.0931)
  line L567 (-1620.0937, 433.1995) -> (-1614.0937, 433.1995)
  line L568 (-1386.4448, 151.4222) -> (-1387.4867, 157.331)
  line L569 (-1393.9133, -62.487) -> (-1399.8222, -63.5289)
  line L570 (-1192.9109, -242.5837) -> (-1192.8646, -237.9663)
  line L571 (-1620.0937, 365.74) -> (-1614.0937, 365.74)
  line L572 (-1450.0582, 280.2873) -> (-1420.0582, 280.2873)
  line L573 (-1614.0937, 273.2805) -> (-1614.0937, 268.2805)
  line L574 (-1614.0937, 500.659) -> (-1614.0937, 495.659)
  line L575 (-1183.9109, -242.5837) -> (-1183.9109, -262.5837)
  line L576 (-1450.0582, 286.2873) -> (-1450.0582, 280.2873)
  line L577 (-1655.0937, 568.1185) -> (-1620.0937, 568.1185)
  line L578 (-1368.3072, -33.9343) -> (-1368.3072, -28.9343)
  line L579 (-1198.9595, -267.8891) -> (-1192.9597, -267.9437)
  line L580 (-1450.0582, 280.2873) -> (-1420.0582, 280.2873)
  line L581 (-1605.0937, 273.2805) -> (-1614.0937, 273.2805)
  line L582 (-1614.0937, 360.74) -> (-1605.0937, 360.74)
  line L583 (-1233.3072, 178.4245) -> (-1252.465, 175.0465) construction
  line L584 (-1228.3072, -127.5755) -> (-1263.3072, -127.5755)
  line L585 (-1368.3072, -60.6009) -> (-1368.3072, -55.6009)
  line L586 (-1299.8388, 172.7857) -> (-1278.173, 176.606)
  line L587 (-1620.0937, 500.659) -> (-1614.0937, 500.659)
  line L588 (-1233.3072, 178.4245) -> (-1430.2687, 143.6949)
  line L589 (-1183.9109, -182.5837) -> (-1183.9109, -202.5837)
  line L590 (-1198.9109, -177.5837) -> (-1198.9109, -171.5837)
  line L591 (-1183.9109, -302.5837) -> (-1183.9109, -322.5837)
  line L592 (-1640.0937, 374.0931) -> (-1640.0937, 369.0931)
  line L593 (-1605.0937, 475.659) -> (-1614.0937, 475.659)
  line L594 (-1614.0937, 568.1185) -> (-1614.0937, 563.1185)
  line L595 (-1450.0582, 286.2873) -> (-1450.0582, 280.2873)
  line L596 (-1192.8541, -178.0547) -> (-1198.9109, -178.0547)
  line L597 (-1605.0937, 495.659) -> (-1605.0937, 475.659)
  line L598 (-1270.0582, 280.2873) -> (-1240.0582, 280.2873)
  line L599 (-1630.0937, 574.1185) -> (-1630.0937, 568.1185)
  line L600 (-1270.0582, 286.2873) -> (-1270.0582, 280.2873)
  line L601 (-1343.6627, 165.0584) -> (-1321.997, 168.8786)
  line L602 (-1821.6086, 326.1651) -> (-1828.5546, 365.5574)
  line L603 (-1360.0582, 280.2873) -> (-1360.0582, 286.2873)
  line L604 (-1192.9597, -267.9437) -> (-1192.9109, -262.5837)
  line L605 (-1645.0937, 574.1185) -> (-1630.0937, 574.1185)
  line L606 (-1192.9714, -208.0216) -> (-1192.9109, -202.5837)
  line L607 (-1605.0937, 563.1185) -> (-1605.0937, 543.1185)
  line L608 (-1192.3306, -96.4119) -> (-1192.3306, -91.4119)
  line L609 (-1192.3072, -53.9523) -> (-1192.3306, -48.9524)
  line L610 (-1198.9109, -507.5837) -> (-1198.9109, -513.5837)
  line L611 (-1192.8718, -297.9053) -> (-1198.9109, -297.9053)
  line L612 (-1228.9109, -177.5837) -> (-1228.9109, -171.5837)
  line L613 (-1676.7594, 564.2983) -> (-1677.8013, 570.2071)
  line L614 (-1270.0582, 286.2873) -> (-1270.0582, 280.2873)
  line L615 (-1775.2809, 262.1185) -> (-1740.2809, 262.1185)
  line L616 (-1270.0582, 280.2873) -> (-1240.0582, 280.2873)
  line L617 (-1240.0582, 280.2873) -> (-1240.0582, 286.2873)
  circle A8 centre (-1095.5897, -121.0941) radius 10
  line L618 (-1270.0582, 280.2873) -> (-1240.0582, 280.2873)
  point P0 (-1910.457, -232.1266)
  point P1 (-1910.457, -232.1266)
  point P2 (-1910.457, -232.1266)
  point P3 (-1910.457, -232.1266)
  point P4 (-1910.457, -232.1266)
  point P5 (-1910.457, -232.1266)
  point P6 (-1910.457, -232.1266)
  point P7 (-1910.457, -232.1266)
  point P8 (-1910.457, -232.1266)
  point P9 (-1910.457, -232.1266)
  point P10 (-1910.457, -232.1266)
  point P11 (-1910.457, -232.1266)
  point P12 (-1243.0582, 486.2873)
  point P13 (-1361.5582, 486.2873)
  point P14 (-1302.3082, 486.2873)
  point P15 (-1315.0435, 486.2902)
  point P16 (-1150.0582, 441.954)
  point P17 (-1232.2747, 286.2873)
  point P18 (-1420.0582, 286.2873)
  point P19 (-1420.0582, 286.2873)
  point P20 (-1420.0582, 286.2873)
  point P21 (-1420.8082, 486.2873)
  point P22 (-1365.4747, 486.2902)
  point P23 (-1240.8082, 286.2873)
  point P24 (-1300.0582, 286.2873)
  point P25 (-1304.7247, 286.2844)
  point P26 (-1192.3192, 286.2844)
  point P27 (-1240.0582, 286.2873)
  point P28 (-1360.8082, 286.2873)
  point P29 (-1240.0582, 286.2873)
  point P30 (-1246.9747, 486.2902)
  point P31 (-1312.3192, 286.2844)
  point P32 (-1192.3192, 286.2844)
  point P33 (-1300.0582, 286.2873)
  point P34 (-1192.3192, 286.2844)
  point P35 (-1412.2747, 286.2873)
  point P36 (-1292.2747, 286.2873)
  point P37 (-1372.3192, 286.2844)
  point P38 (-1480.0582, 317.0669)
  point P39 (-1304.7247, 286.2844)
  point P40 (-1412.2747, 286.2873)
  point P41 (-1192.3192, 286.2844)
  point P42 (-1180.8082, 286.2873)
  point P43 (-1180.8082, 286.2873)
  point P44 (-1244.7247, 286.2844)
  point P45 (-1300.8082, 286.2873)
  point P46 (-1192.3192, 286.2844)
  point P47 (-1172.2747, 286.2873)
  point P48 (-1232.2747, 286.2873)
  point P49 (-1424.7247, 286.2844)
  point P50 (-1172.2747, 286.2873)
  point P51 (-1480.0582, 406.0669)
  point P52 (-1232.2747, 286.2873)
  point P53 (-1232.2747, 286.2873)
  point P54 (-1292.2747, 286.2873)
  point P55 (-1184.7247, 286.2844)
  point P56 (-1244.7247, 286.2844)
  point P57 (-1172.2747, 286.2873)
  point P58 (-1372.3192, 286.2844)
  point P59 (-1252.3192, 286.2844)
  point P60 (-1352.2747, 286.2873)
  point P61 (-1192.3192, 286.2844)
  point P62 (-1252.3192, 286.2844)
  point P63 (-1240.0582, 286.2873)
  point P64 (-1184.7247, 286.2844)
  point P65 (-1240.8082, 286.2873)
  point P66 (-1244.7247, 286.2844)
  point P67 (-1180.8082, 286.2873)
  point P68 (-1300.8082, 286.2873)
  point P69 (-1364.7247, 286.2844)
  point P70 (-1244.7247, 286.2844)
  point P71 (-1240.8082, 286.2873)
  point P72 (-1372.3192, 286.2844)
  point P73 (-1360.0582, 286.2873)
  point P74 (-1360.8082, 286.2873)
  point P75 (-1172.2747, 286.2873)
  point P76 (-1240.0582, 286.2873)
  point P77 (-1300.8082, 286.2873)
  point P78 (-1412.2747, 286.2873)
  point P79 (-1184.7247, 286.2844)
  point P80 (-1304.7247, 286.2844)
  point P81 (-1352.2747, 286.2873)
  point P82 (-1300.0582, 286.2873)
  point P83 (-1372.3192, 286.2844)
  point P84 (-1412.2747, 286.2873)
  point P85 (-1292.2747, 286.2873)
  point P86 (-1312.3192, 286.2844)
  point P87 (-1172.2747, 286.2873)
  point P88 (-1254.5692, 486.2902)
  point P89 (-1432.3192, 486.2902)
  point P90 (-1292.2747, 286.2873)
  point P91 (-1187.7247, 486.2902)
  point P92 (-1373.0692, 486.2902)
  point P93 (-1234.5247, 486.2873)
  point P94 (-1424.7247, 486.2902)
  point P95 (-1353.0247, 486.2873)
  point P96 (-1432.3192, 286.2844)
  point P97 (-1384.0979, -297.5837)
  point P98 (-1384.0979, -417.5837)
  point P99 (-1424.7247, 286.2844)
  point P100 (-1252.3192, 286.2844)
  point P101 (-1240.8082, 286.2873)
  point P102 (-1240.0582, 286.2873)
  point P103 (-1233.6598, -121.0652)
  point P104 (-1244.7247, 286.2844)
  point P105 (-1252.3192, 286.2844)
  point P106 (-1384.0979, -237.5837)
  point P107 (-1384.0979, -237.5837)
  point P108 (-1300.8082, 286.2873)
  point P109 (-1300.0582, 286.2873)
  point P110 (-1360.0582, 286.2873)
  point P111 (-1364.7247, 286.2844)
  point P112 (-1372.3192, 286.2844)
  point P113 (-1184.7247, 286.2844)
  point P114 (-1232.2747, 286.2873)
  point P115 (-1352.2747, 286.2873)
  point P116 (-1312.3192, 286.2844)
  point P117 (-1364.7247, 286.2844)
  point P118 (-1180.8082, 286.2873)
  point P119 (-1384.0979, -357.5837)
  point P120 (-1360.0582, 286.2873)
  point P121 (-1306.2247, 486.2902)
  point P122 (-1313.8192, 486.2902)
  point P123 (-1195.3192, 486.2902)
  point P124 (-1420.8082, 286.2873)
  point P125 (-1312.3192, 286.2844)
  point P126 (-1150.0582, 353.2873)
  point P127 (-1252.3192, 286.2844)
  point P128 (-1360.8082, 286.2873)
  point P129 (-1240.8082, 286.2873)
  point P130 (-1252.3192, 286.2844)
  point P131 (-1315.0435, 286.2844)
  point P132 (-1240.8082, 286.2873)
  point P133 (-1420.8082, 286.2873)
  point P134 (-1240.0582, 286.2873)
  point P135 (-1352.2747, 286.2873)
  point P136 (-1180.8082, 286.2873)
  point P137 (-1420.8082, 286.2873)
  point P138 (-1420.0582, 286.2873)
  point P139 (-1384.0979, -417.5837)
  point P140 (-1420.0582, 286.2873)
  point P141 (-1315.0435, 286.2844)
  point P142 (-1424.7247, 286.2844)
  point P143 (-1432.3192, 286.2844)
  point P144 (-1304.7247, 286.2844)
  point P145 (-1432.3192, 286.2844)
  point P146 (-1180.8082, 286.2873)
  point P147 (-1240.0582, 286.2873)
  point P148 (-1312.3192, 286.2844)
  point P149 (-1480.5265, 406.0674)
  point P150 (-1232.2747, 286.2873)
  point P151 (-1360.8082, 286.2873)
  point P152 (-1232.2747, 286.2873)
  point P153 (-1172.2747, 286.2873)
  point P154 (-1293.7747, 486.2873)
  point P155 (-1471.5247, 486.2873)
  point P156 (-1180.8082, 286.2873)
  point P157 (-1384.0979, -357.5837)
  point P158 (-1384.0979, -297.5837)
  point P159 (-1412.2747, 286.2873)
  point P160 (-1420.8082, 286.2873)
  point P161 (-1360.0582, 286.2873)
  point P162 (-1420.8082, 286.2873)
  point P163 (-1420.8082, 286.2873)
  point P164 (-1312.3192, 286.2844)
  point P165 (-1424.7247, 286.2844)
  point P166 (-1424.7247, 286.2844)
  point P167 (-1412.2747, 286.2873)
  point P168 (-1304.7247, 286.2844)
  point P169 (-1149.1192, 450.5833)
  point P170 (-1432.3192, 286.2844)
  point P171 (-1352.2747, 286.2873)
  point P172 (-1300.8082, 286.2873)
  point P173 (-1252.3192, 286.2844)
  point P174 (-1364.7247, 286.2844)
  point P175 (-1360.0582, 286.2873)
  point P176 (-1292.2747, 286.2873)
  point P177 (-1184.7247, 286.2844)
  point P178 (-1240.8082, 286.2873)
  point P179 (-1300.0582, 286.2873)
  point P180 (-1420.0582, 286.2873)
  point P181 (-1244.7247, 286.2844)
  point P182 (-1412.2747, 486.2873)
  point P183 (-1240.8082, 286.2873)
  point P184 (-1424.7247, 286.2844)
  point P185 (-1432.3192, 286.2844)
  point P186 (-1244.7247, 286.2844)
  point P187 (-1240.0582, 286.2873)
  point P188 (-1172.2747, 286.2873)
  point P189 (-1432.3192, 286.2844)
  point P190 (-1420.0582, 286.2873)
  point P191 (-1352.2747, 286.2873)
  point P192 (-1150.0582, 353.2873)
  point P193 (-1150.0582, 397.6206)
  point P194 (-1149.1192, 317.5833)
  point P195 (-1150.0582, 441.954)
  point P196 (-1150.0582, 397.6206)
  point P197 (-1655.4463, 268.6288)
  point P198 (-1669.6252, 451.2878)
  point P199 (-1149.1192, 406.2499)
  point P200 (-1149.1192, 361.9166)
  point P201 (-1480.5265, 361.5674)
  point P202 (-1292.2747, 286.2873)
  point P203 (-1300.0582, 286.2873)
  point P204 (-1480.5265, 317.0674)
  point P205 (-1247.8387, 61.5938)
  point P206 (-1432.3192, 286.2844)
  point P207 (-1420.8082, 286.2873)
  point P208 (-1360.0582, 286.2873)
  point P209 (-1300.8082, 286.2873)
  point P210 (-1352.2747, 286.2873)
  point P211 (-1300.0582, 286.2873)
  point P212 (-1412.2747, 286.2873)
  point P213 (-1432.3192, 286.2844)
  point P214 (-1292.2747, 286.2873)
  point P215 (-1372.3192, 286.2844)
  point P216 (-1360.8082, 286.2873)
  point P217 (-1364.7247, 286.2844)
  point P218 (-1360.8082, 286.2873)
  point P219 (-1252.3192, 286.2844)
  point P220 (-1304.7247, 286.2844)
  point P221 (-1372.3192, 286.2844)
  point P222 (-1364.7247, 286.2844)
  point P223 (-1480.5265, 450.5674)
  point P224 (-1172.2747, 286.2873)
  point P225 (-1312.3192, 286.2844)
  point P226 (-1300.8082, 286.2873)
  point P227 (-1304.7247, 286.2844)
  point P228 (-1420.0582, 286.2873)
  point P229 (-1360.8082, 286.2873)
  point P230 (-1300.0582, 286.2873)
  point P231 (-1315.0435, 286.2844)
  point P232 (-1424.7247, 286.2844)
  point P233 (-1184.7247, 286.2844)
  point P234 (-1352.2747, 286.2873)
  point P235 (-1300.8082, 286.2873)
  point P236 (-1292.2747, 286.2873)
  point P237 (-1192.3192, 286.2844)
  point P238 (-1424.7247, 286.2844)
  point P239 (-1480.0582, 361.5669)
  point P240 (-1420.8082, 286.2873)
  point P241 (-1360.0582, 286.2873)
  point P242 (-1312.3192, 286.2844)
  point P243 (-1364.7247, 286.2844)
  point P244 (-1360.0582, 286.2873)
  point P245 (-1192.3192, 286.2844)
  point P246 (-1364.7247, 286.2844)
  point P247 (-1247.8387, 61.5938)
  point P248 (-1372.3192, 286.2844)
  point P249 (-1304.7247, 286.2844)
  point P250 (-1184.7247, 286.2844)
  point P251 (-1184.7247, 286.2844)
  point P252 (-1232.2747, 286.2873)
  point P253 (-1360.8082, 286.2873)
  point P254 (-1180.8082, 286.2873)
  point P255 (-1412.2747, 286.2873)
  point P256 (-1244.7247, 286.2844)
  point P257 (-1221.7576, 486.2873)
  dimension "d1" = 269.363
  dimension "d2" = 330
  dimension "d3" = 40
  dimension "d4" = 165
  dimension "d5" = 165
  dimension "d6" = 30
  dimension "d7" = 6
  dimension "d8" = 6
  dimension "d9" = 6
  dimension "d10" = 6
  dimension "d11" = 6
  dimension "d12" = 6
  dimension "d13" = 6
  dimension "d14" = 30
  dimension "d15" = 6
  dimension "d16" = 6
  dimension "d17" = 6
  dimension "d18" = 6
  dimension "d19" = 6
  dimension "d20" = 6
  dimension "d21" = 6
  dimension "d22" = 6
  dimension "d23" = 6
  dimension "d24" = 6
  dimension "d25" = 6
  dimension "d26" = 6
  dimension "d27" = 6
  dimension "d28" = 6
  dimension "d29" = 6
  dimension "d30" = 6
  dimension "d31" = 6
  dimension "d32" = 6
  dimension "d33" = 6
  dimension "d34" = 6
  dimension "d35" = 6
  dimension "d36" = 6
  dimension "d37" = 6
  dimension "d38" = 6
  dimension "d39" = 6
  dimension "d40" = 6
  dimension "d41" = 6
  dimension "d42" = 6
  dimension "d43" = 269.363
  dimension "d44" = 330
  dimension "d45" = 40
  dimension "d46" = 165
  dimension "d47" = 165
  dimension "d48" = 30
  dimension "d49" = 6
  dimension "d50" = 6
  dimension "d51" = 6
  dimension "d52" = 6
  dimension "d53" = 6
  dimension "d54" = 6
  dimension "d55" = 6
  dimension "d56" = 30
  dimension "d57" = 6
  dimension "d58" = 6
  dimension "d59" = 6
  dimension "d60" = 6
  dimension "d61" = 6
  dimension "d62" = 6
  dimension "d63" = 6
  dimension "d64" = 6
  dimension "d65" = 6
  dimension "d66" = 6
  dimension "d67" = 6
  dimension "d68" = 6
  dimension "d69" = 6
  dimension "d70" = 6
  dimension "d71" = 6
  dimension "d72" = 6
  dimension "d73" = 6
  dimension "d74" = 6
  dimension "d75" = 6
  dimension "d76" = 6
  dimension "d77" = 6
  dimension "d78" = 6
  dimension "d79" = 6
  dimension "d80" = 6
  dimension "d81" = 6
  dimension "d82" = 6
  dimension "d83" = 6
  dimension "d84" = 6
  dimension "d85" = 269.363
  dimension "d86" = 330
  dimension "d87" = 40
  dimension "d88" = 165
  dimension "d89" = 165
  dimension "d90" = 30
  dimension "d91" = 6
  dimension "d92" = 6
  dimension "d93" = 6
  dimension "d94" = 6
  dimension "d95" = 6
  dimension "d96" = 6
  dimension "d97" = 6
  dimension "d98" = 30
  dimension "d99" = 6
  dimension "d100" = 6
  dimension "d101" = 6
  dimension "d102" = 6
  dimension "d103" = 6
  dimension "d104" = 6
  dimension "d105" = 6
  dimension "d106" = 6
  dimension "d107" = 6
  dimension "d108" = 6
  dimension "d109" = 6
  dimension "d110" = 6
  dimension "d111" = 6
  dimension "d112" = 6
  dimension "d113" = 6
  dimension "d114" = 6